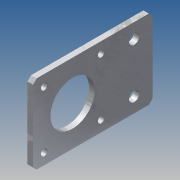
# Autodesk Inventor part: Nema17_Montageplatte_Extruder
Saved by Autodesk Inventor 2015 SP1 (Build 190203100, 203)
## iProperties
Created: 2015-01-06
Part Number: Nema17_Montageplatte_Extruder
Material: Aluminium 6061
Document SubType Name: Modeling
Designer: Marc
Density: 2.7 g/cm^3
Appearance: Aluminium - flach
Mass: 21.42 g
Surface Area: 62.3386 cm^2
Volume: 7.93335 cm^3
Author: Marc
Autodesk Inventor part; units mm, degrees
ref_plane "YZ Plane" through (0, 0, 0) normal (1, 0, 0) x (0, 1, 0)
ref_plane "XZ Plane" through (0, 0, 0) normal (0, 1, 0) x (-1, 0, 0)
ref_plane "XY Plane" through (0, 0, 0) normal (0, 0, 1) x (1, 0, 0)
sketch "Skizze1" plane through (0, 0, 0) normal (1, 0, 0) x (0, 1, 0)
  line L0 (0, -30.1) -> (0, 30.1) projected
  line L1 (-45.5, 0) -> (45.5, 0) projected
  line L2 (-30.5, 21.5) -> (30.5, 21.5)
  line L3 (32.5, 19.5) -> (32.5, -19.5)
  line L4 (30.5, -21.5) -> (-30.5, -21.5)
  line L5 (-32.5, -19.5) -> (-32.5, 19.5)
  circle A0 centre (22.5, 13.5) radius 2.75
  circle A1 centre (22.5, -13.5) radius 2.75
  line L6 (30.5, 21.5) -> (32.5, 19.5)
  line L7 (32.5, -19.5) -> (30.5, -21.5)
  line L8 (-30.5, 21.5) -> (-32.5, 19.5)
  line L9 (-30.5, -21.5) -> (-32.5, -19.5)
  circle A2 centre (-11, 0) radius 12
  circle A3 centre (-26.5, 15.5) radius 1.75
  circle A4 centre (-26.5, -15.5) radius 1.75
  circle A5 centre (4.5, 15.5) radius 1.75
  circle A6 centre (4.5, -15.5) radius 1.75
  point P0 (0, 0)
  point P1 (-32.5, 21.5)
  point P2 (32.5, -21.5)
  point P3 (32.5, 21.5)
  point P4 (-32.5, -21.5)
  dimension "d0" = 65
  dimension "d1" = 43
  dimension "d2" = 5.5
  dimension "d3" = 10
  dimension "d4" = 8
  dimension "d14" = 2
  dimension "d15" = 2
  dimension "d16" = 2
  dimension "d17" = 2
  dimension "d18" = 2
  dimension "d19" = 2
  dimension "d20" = 2
  dimension "d21" = 2
  dimension "d35" = 24
  dimension "d43" = 3.5
  dimension "d44" = 15.5
  dimension "d46" = 15.5
  dimension "d47" = 21.5
  dimension "d48" = 3.5
  dimension "d49" = 15.5
  dimension "d50" = 15.5
  constraints: 16 end point, 9 point on line, 7 centre point, 3 symmetric about line, 2 parallel, 1 horizontal, 1 perpendicular, 5 other
  measures "d0" distance of point (32.5, -21.5) point (-32.5, -21.5)
  measures "d1" distance of point (32.5, 21.5) point (32.5, -21.5)
  measures "d2" diameter of A0
  measures "d3" distance from line of L3 A0.centre
  measures "d4" distance from line of L2 A0.centre
  measures "d14" distance of L2.end point (32.5, 21.5)
  measures "d15" distance of L3.start point (32.5, 21.5)
  measures "d16" distance of L3.end point (32.5, -21.5)
  measures "d17" distance of L4.start point (32.5, -21.5)
  measures "d18" distance of L2.start point (-32.5, 21.5)
  measures "d19" distance of L5.end point (-32.5, 21.5)
  measures "d20" distance of L4.end point (-32.5, -21.5)
  measures "d21" distance of L5.start point (-32.5, -21.5)
  measures "d35" diameter of A2
  measures "d43" diameter of A3
  measures "d44" distance from line of L1 A3.centre
  measures "d46" horizontal distance of A2.centre A3.centre
  measures "d47" distance from line of L5 A2.centre
  measures "d48" diameter of A5
  measures "d49" distance from line of L1 A5.centre
  measures "d50" horizontal distance of A2.centre A5.centre
extrude "Extrusion5" add sketch "Skizze1" along normal blind 3 contours L4 L9 L5 L1 A2 L0 | L0 A2 L1 L3 L7 L4 | L1 L5 L8 L2 L0 A2 | A2 L0 L2 L6 L3 L1
equation "\"d15\" = d14"
equation "\"d16\" = d14"
equation "\"d17\" = d16"
equation "\"d18\" = d14"
equation "\"d19\" = d18"
equation "\"d20\" = d14"
equation "\"d21\" = d20"
